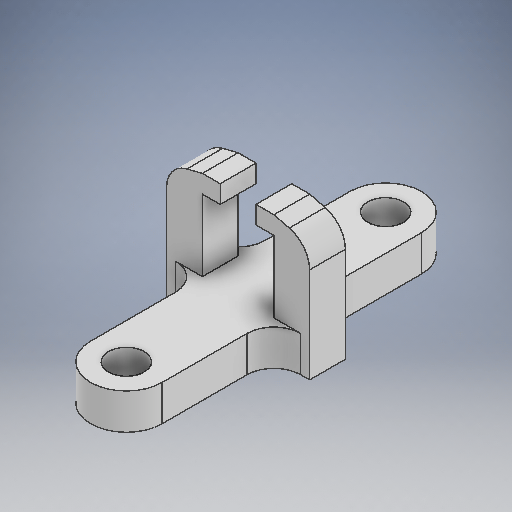
# Autodesk Inventor part: leg_wire_holder
Saved by Autodesk Inventor 2026.1 (Build 301233000, 233)
## iProperties
Created: 2025-12-05
Part Number: leg_wire_holder
Material: Generic
Document SubType Name: Modeling
Designer: emanuel
Density: 1 g/cm^3
Appearance: Default
Author: emanuel
Autodesk Inventor part; units mm, degrees
ref_plane "YZ Plane" through (0, 0, 0) normal (1, 0, 0) x (0, 1, 0)
ref_plane "XZ Plane" through (0, 0, 0) normal (0, 1, 0) x (-1, 0, 0)
ref_plane "XY Plane" through (0, 0, 0) normal (0, 0, 1) x (1, 0, 0)
sketch "Sketch1" plane through (0, 0, 0) normal (0, 1, 0) x (-1, 0, 0)
  circle A0 centre (0, 0) radius 1
  circle A1 centre (0, 0) radius 2
  line L0 (2, 0) -> (-2, 0)
  line L1 (-2, 0) -> (-2, -8.25)
  line L2 (-2, -8.25) -> (2, -8.25)
  line L3 (2, -8.25) -> (2, 0)
  line L4 (2, -8.25) -> (4, -8.25)
  line L5 (4, -8.25) -> (4, -6.25)
  line L6 (4, -6.25) -> (2, -6.25)
  line L7 (2, -6.25) -> (2, -8.25)
  line L8 (-2, -8.25) -> (-4, -8.25)
  line L9 (-4, -8.25) -> (-4, -6.25)
  line L10 (-4, -6.25) -> (-2, -6.25)
  line L11 (-2, -6.25) -> (-2, -8.25)
  line L12 (0, 0) -> (0, -14.5)
  line L13 (0, 0) -> (14.5, 0) construction
  circle A2 centre (0, -14.5) radius 1
  circle A3 centre (0, -14.5) radius 2
  line L14 (2, -8.25) -> (-2, -8.25)
  line L15 (-2, -8.25) -> (-2, -14.5)
  line L16 (-2, -14.5) -> (2, -14.5)
  line L17 (2, -14.5) -> (2, -8.25)
  point P0 (-2, -6.25)
  point P1 (2, -6.25)
  point P2 (2, -14.5)
  dimension "d1" = 4
  dimension "d25" = 4
  dimension "d0" = 2
  dimension "d2" = 8.25
  dimension "d3" = 2
  dimension "d4" = 2
  dimension "d5" = 2
  dimension "d6" = 2
  dimension "d22" = 14.5
  dimension "d23" = 90
  dimension "d24" = 2
  constraints: 36 end point, 8 parallel, 5 horizontal, 5 perpendicular, 4 coincident, 2 centre point, 1 vertical, 6 other
  measures "d0" diameter of A0
  measures "d2" distance of L1.end L0.end
  measures "d3" distance of L6.end L5.end
  measures "d4" distance of L5.end L4.end
  measures "d5" distance of L9.end L10.end
  measures "d6" distance of L8.end L9.end
  measures "d22" distance of L12.start L12.end
  measures "d23" angle of L12 L13
  measures "d24" diameter of A2
extrude "Extrusion1" add sketch "Sketch1" along normal blind 2 contours L0 A1 L12 A0 | A0 L0 A1 | A0 L12 A1 L0 | L3 L2 L12 A1 | A1 L12 L2 L1 | L6 L5 L4 L3 | L1 L8 L9 L10 | L12 A3 L15 L2 | L2 L17 A3 L12 | A3 L16 A2 L12 | L12 A2 L16 A3 | A3 L16 A2
sketch "Sketch2" plane through (0, 2, 0) normal (0, 1, 0) x (1, 0, 0)
  line L0 (-4, 6.25) -> (-2, 6.25) projected
  line L1 (4, 8.25) -> (-4, 8.25) projected
  line L2 (-4, 6.25) -> (-2, 6.25)
  line L3 (-2, 6.25) -> (-2, 8.25)
  line L4 (-2, 8.25) -> (-4, 8.25)
  line L5 (-4, 8.25) -> (-4, 6.25)
  line L6 (4, 6.25) -> (2, 6.25)
  line L7 (2, 6.25) -> (2, 8.25)
  line L8 (2, 8.25) -> (4, 8.25)
  line L9 (4, 8.25) -> (4, 6.25)
  point P0 (0, 0)
  point P1 (-4, 8.25)
  point P2 (-2, 6.25)
  dimension "d9" = 2
  dimension "d10" = 2
  constraints: 16 end point, 4 parallel, 3 point on line, 2 horizontal, 2 perpendicular
  measures "d9" distance of L4.end L3.end
  measures "d10" distance of L7.end L8.end
extrude "Extrusion2" add sketch "Sketch2" along normal blind 4.5
sketch "Sketch3" plane through (4, 0, -8.25) normal (0, 0, -1) x (-1, 0, 0)
  line L0 (2, 6.5) -> (0, 6.5) projected
  line L1 (2, 6.5) -> (2, 6)
  line L2 (2, 2) -> (2, 6.5) projected
  line L3 (2, 6) -> (6, 6)
  line L4 (2, 6) -> (3, 6)
  line L5 (3, 6) -> (3, 7)
  line L6 (3, 7) -> (2, 7)
  line L7 (2, 7) -> (2, 6)
  line L8 (6, 6) -> (5, 6)
  line L9 (5, 6) -> (5, 7)
  line L10 (5, 7) -> (6, 7)
  line L11 (6, 7) -> (6, 6)
  line L12 (2, 7) -> (0, 6.5)
  line L13 (8, 0) -> (8, 6.5) projected
  line L14 (6, 7) -> (8, 6.5)
  line L15 (8, 6.5) -> (6, 6.5)
  line L16 (0, 6.5) -> (2, 6.5)
  point P0 (4, 0)
  dimension "d13" = 0.5
  dimension "d14" = 4
  dimension "d15" = 1
  dimension "d16" = 1
  dimension "d17" = 1
  dimension "d18" = 1
  constraints: 28 end point, 4 parallel, 3 perpendicular, 2 horizontal, 1 midpoint, 1 point on line
  measures "d13" distance of L0.start L1.end
  measures "d14" distance of L1.end L3.end
  measures "d15" distance of L6.end L5.end
  measures "d16" distance of L5.end L4.end
  measures "d17" distance of L9.end L10.end
  measures "d18" distance of L8.end L9.end
extrude "Extrusion3" add sketch "Sketch3" against normal blind 2
fillet "Fillet1" radius 1.5 2 edges at (4, 6.5, -7.25) (-4, 6.5, -7.25)
fillet "Fillet2" radius 1.5 4 edges at (-2, 1, -6.25) (2, 1, -6.25) (-2, 1, -8.25) (2, 1, -8.25)
body "Solid1"
